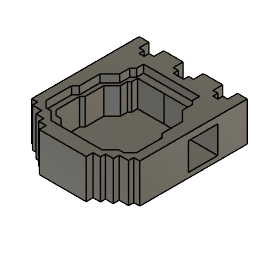
Fantasma PacMan (f3d) (Autodesk Fusion 360 design; units mm, degrees)
part number: 2026-06-05-10-05-34-464
Autodesk Fusion 360 part; units mm, degrees
sketch "Boceto1" plane through (0, 0, 0) normal (0, 0, 1) x (1, 0, 0)
  line L0 (0, 0) -> (0, 10) construction
  line L1 (55.2426, -86.6569) -> (49.1066, -86.6569)
  line L2 (0, -110.0711) -> (24, -110.0711)
  line L3 (24, -110.0711) -> (24, -103.0711)
  line L4 (24, -103.0711) -> (31.5563, -103.0711)
  line L5 (31.5563, -103.0711) -> (31.5563, -97.935)
  line L6 (31.5563, -97.935) -> (39.5563, -97.935)
  line L7 (39.5563, -97.935) -> (39.5563, -91.935)
  line L8 (39.5563, -91.935) -> (49.1066, -91.935)
  line L9 (49.1066, -91.935) -> (49.1066, -86.6569)
  line L10 (55.2426, -86.6569) -> (55.2426, 23.3431)
  line L11 (55.2426, 23.3431) -> (45.2426, 23.3431)
  line L12 (45.2426, 23.3431) -> (45.2426, 13.3431)
  line L13 (45.2426, 13.3431) -> (40.2426, 13.3431)
  line L14 (40.2426, 13.3431) -> (40.2426, 8.3431)
  line L15 (40.2426, 8.3431) -> (35.2426, 8.3431)
  line L16 (35.2426, 8.3431) -> (35.2426, 13.3431)
  line L17 (35.2426, 13.3431) -> (30.2426, 13.3431)
  line L18 (30.2426, 13.3431) -> (30.2426, 23.3431)
  line L19 (30.2426, 23.3431) -> (10.2426, 23.3431)
  line L20 (10.2426, 23.3431) -> (10.2426, 13.3431)
  line L21 (10.2426, 13.3431) -> (5.2426, 13.3431)
  line L22 (5.2426, 13.3431) -> (5.2426, 8.3431)
  line L23 (5.2426, 8.3431) -> (0, 8.3431)
  line L24 (0, -110.0711) -> (-24, -110.0711)
  line L25 (-24, -110.0711) -> (-24, -103.0711)
  line L26 (-24, -103.0711) -> (-31.5563, -103.0711)
  line L27 (-31.5563, -103.0711) -> (-31.5563, -97.935)
  line L28 (-31.5563, -97.935) -> (-39.5563, -97.935)
  line L29 (-39.5563, -97.935) -> (-39.5563, -91.935)
  line L30 (-39.5563, -91.935) -> (-49.1066, -91.935)
  line L31 (-49.1066, -91.935) -> (-49.1066, -86.6569)
  line L32 (-55.2426, -86.6569) -> (-49.1066, -86.6569)
  line L33 (-55.2426, -86.6569) -> (-55.2426, 23.3431)
  line L34 (-55.2426, 23.3431) -> (-45.2426, 23.3431)
  line L35 (-45.2426, 23.3431) -> (-45.2426, 13.3431)
  line L36 (-45.2426, 13.3431) -> (-40.2426, 13.3431)
  line L37 (-40.2426, 13.3431) -> (-40.2426, 8.3431)
  line L38 (-40.2426, 8.3431) -> (-35.2426, 8.3431)
  line L39 (-35.2426, 8.3431) -> (-35.2426, 13.3431)
  line L40 (-35.2426, 13.3431) -> (-30.2426, 13.3431)
  line L41 (-30.2426, 13.3431) -> (-30.2426, 23.3431)
  line L42 (-30.2426, 23.3431) -> (-10.2426, 23.3431)
  line L43 (-10.2426, 23.3431) -> (-10.2426, 13.3431)
  line L44 (-10.2426, 13.3431) -> (-5.2426, 13.3431)
  line L45 (-5.2426, 13.3431) -> (-5.2426, 8.3431)
  line L46 (-5.2426, 8.3431) -> (0, 8.3431)
  line L47 (-40.4532, -52.2423) -> (-36.5208, -52.2423) construction
  line L48 (-0.0272, -88.2631) -> (-23.5522, -88.2903)
  line L49 (-23.5522, -88.2903) -> (-30.6587, -81.1839)
  line L50 (-23.5522, -88.2903) -> (-13.5022, -88.2903) construction
  line L51 (-30.6587, -81.1839) -> (-35.7087, -81.1839)
  line L52 (-35.7087, -81.1839) -> (-40.6938, -76.1988)
  line L53 (-35.7087, -81.1839) -> (-28.6587, -81.1839) construction
  line L54 (-40.6938, -76.1988) -> (-40.6938, -52.1488)
  line L55 (-40.6938, -52.1488) -> (-37.83, -49.285)
  line L56 (-40.6938, -52.1488) -> (-36.6438, -52.1488) construction
  line L57 (-37.83, -49.285) -> (-37.83, -30.235)
  line L58 (-37.83, -30.235) -> (-29.3093, -21.7144)
  line L59 (-37.83, -30.235) -> (-25.78, -30.235) construction
  line L60 (-29.3093, -21.7144) -> (-29.3093, -14.6644)
  line L61 (-29.3093, -14.6644) -> (-27.1527, -12.5077)
  line L62 (-29.3093, -14.6644) -> (-26.2593, -14.6644) construction
  line L63 (-27.1527, -12.5077) -> (-27.1527, -6.4577)
  line L64 (-0.0272, -88.2631) -> (-0.0272, -6.4263) construction
  line L65 (-0.0272, -6.4263) -> (-27.1527, -6.4577)
  line L66 (-0.0272, -88.2631) -> (23.4977, -88.2903)
  line L67 (23.4977, -88.2903) -> (30.6042, -81.1839)
  line L68 (30.6042, -81.1839) -> (35.6542, -81.1839)
  line L69 (35.6542, -81.1839) -> (40.6393, -76.1988)
  line L70 (40.6393, -76.1988) -> (40.6393, -52.1488)
  line L71 (40.6393, -52.1488) -> (37.7755, -49.285)
  line L72 (37.7755, -49.285) -> (37.7755, -30.235)
  line L73 (37.7755, -30.235) -> (29.2548, -21.7144)
  line L74 (29.2548, -21.7144) -> (29.2548, -14.6644)
  line L75 (29.2548, -14.6644) -> (27.0982, -12.5077)
  line L76 (27.0982, -12.5077) -> (27.0982, -6.4577)
  line L77 (-0.0272, -6.4263) -> (27.0982, -6.4577)
  line L78 (0, -96.0218) -> (0, 0.9507) construction
  line L79 (0, -96.0218) -> (-25.935, -96.0218)
  line L80 (-25.935, -96.0218) -> (-34.5352, -87.4216)
  line L81 (-25.935, -96.0218) -> (-13.7725, -96.0218) construction
  line L82 (-34.5352, -87.4216) -> (-39.6602, -87.4216)
  line L83 (-39.6602, -87.4216) -> (-46.2203, -80.8614)
  line L84 (-39.6602, -87.4216) -> (-30.3827, -87.4216) construction
  line L85 (-46.2203, -80.8614) -> (-46.2203, -54.8264)
  line L86 (-46.2203, -54.8264) -> (-42.2102, -50.8163)
  line L87 (-46.2203, -54.8264) -> (-40.5491, -54.8264) construction
  line L88 (-42.2102, -50.8163) -> (-42.2102, -29.8813)
  line L89 (-42.2102, -29.8813) -> (-32.08, -19.7511)
  line L90 (-42.2102, -29.8813) -> (-27.8839, -29.8813) construction
  line L91 (-32.08, -19.7511) -> (-32.08, -9.5261)
  line L92 (-32.08, -9.5261) -> (-28.5798, -6.0259)
  line L93 (-32.08, -9.5261) -> (-27.13, -9.5261) construction
  line L94 (-28.5798, -6.0259) -> (-28.5798, 1.1391)
  line L95 (-28.5798, 1.1391) -> (0, 1.1391)
  line L96 (0, -96.0218) -> (25.935, -96.0218)
  line L97 (25.935, -96.0218) -> (34.5352, -87.4216)
  line L98 (34.5352, -87.4216) -> (39.6602, -87.4216)
  line L99 (39.6602, -87.4216) -> (46.2203, -80.8614)
  line L100 (46.2203, -80.8614) -> (46.2203, -54.8264)
  line L101 (46.2203, -54.8264) -> (42.2102, -50.8163)
  line L102 (42.2102, -50.8163) -> (42.2102, -29.8813)
  line L103 (42.2102, -29.8813) -> (32.08, -19.7511)
  line L104 (32.08, -19.7511) -> (32.08, -9.5261)
  line L105 (32.08, -9.5261) -> (28.5798, -6.0259)
  line L106 (28.5798, -6.0259) -> (28.5798, 1.1391)
  line L107 (28.5798, 1.1391) -> (0, 1.1391)
  point P0 (0, 4.7536)
  point P1 (0, 4.7536)
  point P2 (0, 4.7536)
  point P3 (0, -47.5355)
  point P4 (0, 2.3859)
  point P5 (0, 2.3859)
  point P6 (0, 2.3859)
  point P7 (0, -47.5355)
  point P8 (0, 0.9507)
  point P9 (0, -47.5355)
  point P10 (0, 0.9507)
  point P11 (0, -47.5355)
  point P12 (0, 0.9507)
  dimension "d46" = 24
  dimension "d48" = 7
  dimension "d49" = 8
  dimension "d50" = 6
  dimension "d52" = 110
  dimension "d53" = 10
  dimension "d54" = 10
  dimension "d55" = 5
  dimension "d56" = 5
  dimension "d57" = 5
  dimension "d58" = 5
  dimension "d59" = 5
  dimension "d60" = 10
  dimension "d61" = 20
  dimension "d62" = 10
  dimension "d63" = 5
  dimension "d64" = 5
  dimension "d144" = 135
  dimension "d145" = 10.05
  dimension "d146" = 5.05
  dimension "d147" = 135
  dimension "d148" = 7.05
  dimension "d149" = 24.05
  dimension "d150" = 4.05
  dimension "d151" = 45
  dimension "d152" = 19.05
  dimension "d153" = 45
  dimension "d154" = 12.05
  dimension "d155" = 7.05
  dimension "d156" = 3.05
  dimension "d157" = 45
  dimension "d158" = 6.05
  dimension "d168" = 135
  dimension "d169" = 12.1625
  dimension "d171" = 5.125
  dimension "d173" = 135
  dimension "d174" = 9.2775
  dimension "d176" = 26.035
  dimension "d178" = 5.6712
  dimension "d179" = 45
  dimension "d181" = 20.935
  dimension "d183" = 45
  dimension "d184" = 14.3262
  dimension "d186" = 10.225
  dimension "d188" = 4.95
  dimension "d189" = 45
  dimension "d191" = 7.165
  constraint coincident L0.start origin
  constraint coincident P2 P1
  constraint perpendicular L2 L3
  constraint perpendicular L3 L4
  constraint perpendicular L4 L5
  constraint perpendicular L5 L6
  constraint perpendicular L6 L7
  constraint perpendicular L7 L8
  constraint perpendicular L1 L9
  constraint perpendicular L1 L10
  constraint perpendicular L10 L11
  constraint perpendicular L11 L12
  constraint perpendicular L12 L13
  constraint perpendicular L13 L14
  constraint perpendicular L14 L15
  constraint perpendicular L15 L16
  constraint perpendicular L16 L17
  constraint perpendicular L17 L18
  constraint perpendicular L18 L19
  constraint perpendicular L17 L20
  constraint perpendicular L20 L21
  constraint perpendicular L17 L22
  constraint coincident L0 L23.end
  constraint coincident P6 P5
  constraint horizontal L47
  constraint coincident P12 P10
  constraint horizontal L50
  constraint horizontal L51
  constraint horizontal L53
  constraint vertical L54
  constraint horizontal L56
  constraint horizontal L59
  constraint vertical L60
  constraint horizontal L62
  constraint vertical L63
  constraint vertical L64
  constraint coincident L48.start L64.start
  constraint symmetric L48.end L64 L66.end
  constraint symmetric L48.start L64 L66.start
  constraint symmetric L49.end L64 L67.end
  constraint symmetric L51.end L64 L68.end
  constraint symmetric L52.end L64 L69.end
  constraint symmetric L54.end L64 L70.end
  constraint symmetric L55.end L64 L71.end
  constraint symmetric L57.end L64 L72.end
  constraint symmetric L58.end L64 L73.end
  constraint symmetric L60.end L64 L74.end
  constraint symmetric L61.end L64 L75.end
  constraint symmetric L63.end L64 L76.end
  constraint symmetric L65.start L64 L77.start
  constraint perpendicular L78 L79
  constraint horizontal L81
  constraint horizontal L82
  constraint horizontal L84
  constraint vertical L85
  constraint horizontal L87
  constraint vertical L88
  constraint horizontal L90
  constraint vertical L91
  constraint horizontal L93
  constraint vertical L94
  constraint horizontal L95
  constraint coincident L0 L95.end
  constraint perpendicular L0 L95
  constraint symmetric L79.start L78 L96.start
  constraint symmetric L78 L79.end L96.end
  constraint symmetric L78 L80.end L97.end
  constraint symmetric L78 L82.end L98.end
  constraint symmetric L78 L83.end L99.end
  constraint symmetric L78 L85.end L100.end
  constraint symmetric L78 L86.end L101.end
  constraint symmetric L78 L88.end L102.end
  constraint symmetric L78 L89.end L103.end
  constraint symmetric L78 L91.end L104.end
  constraint symmetric L78 L92.end L105.end
  constraint symmetric L78 L94.end L106.end
  constraint symmetric L78 L95.end L107.end
  measures "d46" distance of L2.start L2.end
  measures "d48" distance of L2.end L3.end
  measures "d49" distance of L5.end L6.end
  measures "d50" distance of L6.end L7.end
  measures "d52" distance of L1.start L10.end
  measures "d53" distance of L10.end L11.end
  measures "d54" distance of L11.end L12.end
  measures "d55" distance of L12.end L13.end
  measures "d56" distance of L13.end L14.end
  measures "d57" distance of L14.end L15.end
  measures "d58" distance of L15.end L16.end
  measures "d59" distance of L16.end L17.end
  measures "d60" distance of L17.end L18.end
  measures "d61" distance of L18.end L19.end
  measures "d62" distance of L19.end L20.end
  measures "d63" distance of L20.end L21.end
  measures "d64" distance of L21.end L22.end
  measures "d144" angle of L49 L50
  measures "d145" distance of L48.end L49.end
  measures "d146" distance of L49.end L51.end
  measures "d147" angle of L52 L53
  measures "d148" distance of L51.end L52.end
  measures "d149" distance of L52.end L54.end
  measures "d150" distance of L54.end L55.end
  measures "d151" angle of L55 L56
  measures "d152" distance of L55.end L57.end
  measures "d153" angle of L58 L59
  measures "d154" distance of L57.end L58.end
  measures "d155" distance of L58.end L60.end
  measures "d156" distance of L60.end L61.end
  measures "d157" angle of L61 L62
  measures "d158" distance of L61.end L63.end
  measures "d168" angle of L80 L81
  measures "d169" distance of L79.end L80.end
  measures "d171" distance of L80.end L82.end
  measures "d173" angle of L83 L84
  measures "d174" distance of L82.end L83.end
  measures "d176" distance of L83.end L85.end
  measures "d178" distance of L85.end L86.end
  measures "d179" angle of L86 L87
  measures "d181" distance of L86.end L88.end
  measures "d183" angle of L89 L90
  measures "d184" distance of L88.end L89.end
  measures "d186" distance of L89.end L91.end
  measures "d188" distance of L91.end L92.end
  measures "d189" angle of L92 L93
  measures "d191" distance of L92.end L94.end
ref_plane "PlanoDeObra1" through (55.2426, 23.3431, 35) normal (1, 0, 0) x (0, 1, 0)
sketch "Boceto2" plane through (55.2426, 0, 0) normal (1, 0, 0) x (0, 1, 0)
  line L0 (23.1427, -0.0591) -> (-6.8573, -0.0187)
  line L1 (-6.8573, -0.0187) -> (-6.8573, 32.9813)
  line L2 (-6.8573, 32.9813) -> (-36.8573, 32.9813)
  line L3 (-36.8573, 32.9813) -> (-36.8573, 4.9813)
  line L4 (-36.8573, 4.9813) -> (-6.8573, 4.9813)
  dimension "d198" = 30
  dimension "d200" = 30
  dimension "d201" = 28
  constraint perpendicular L1 L2
  constraint perpendicular L2 L3
  constraint coincident L1 L4.end
  constraint perpendicular L1 L4
  measures "d198" distance of L0.start L0.end
  measures "d200" distance of L1.end L2.end
  measures "d201" distance of L2.end L3.end
extrude "Extruir16" add sketch "Boceto1" along normal blind 5 contours L48 L49 L51 L52 L54 L55 L57 L58 L60 L61 L63 L65 L66 L67 L68 L69 L70 L71 L72 L73 L74 L75 L76 L77
extrude "Extruir17" add sketch "Boceto1" along normal blind 32 contours L79 L80 L82 L83 L85 L86 L88 L89 L91 L92 L94 L95 L96 L97 L98 L99 L100 L101 L102 L103 L104 L105 L106 L107
extrude "Extruir18" add sketch "Boceto1" along normal blind 40 contours L1 L2 L3 L4 L5 L6 L7 L8 L9 L10 L11 L12 L13 L14 L15 L16 L17 L18 L19 L20 L21 L22 L23 L24 L25 L26 L27 L28 L29 L30 L31 L32 L33 L34 L35 L36 L37 L38 L39 L40 L41 L42 L43 L44 L45 L46
extrude "Extruir19" cut sketch "Boceto2" along normal mid plane 60
equation "d169 = 12.13748388 mm + 0.025 mm"
equation "d171 = 5.10 mm + 0.025 mm"
equation "d174 = 9.25248834 mm + 0.025 mm"
equation "d176 = 26.01 mm + 0.025 mm"
equation "d178 = 5.64624366 mm + 0.025 mm"
equation "d181 = 20.91 mm + 0.025 mm"
equation "d184 = 14.3012313 mm + 0.025 mm"
equation "d186 = 10.20 mm + 0.025 mm"
equation "d188 = 4.92499554 mm + 0.025 mm"
equation "d191 = 7.14 mm + 0.025 mm"
